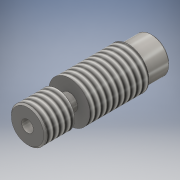
# Autodesk Inventor part: Heatbreak
Saved by Autodesk Inventor 2016 (Build 200138000, 138)
## iProperties
Created: 2016-03-26
Part Number: Heatbreak
Material: Stainless Steel
Document SubType Name: Modeling
Designer: Scott
Density: 8 g/cm^3
Appearance: Semi-Polished
Mass: 5.24058 g
Surface Area: 5.31118 cm^2
Volume: 0.655072 cm^3
Author: Scott
Autodesk Inventor part; units mm, degrees
ref_plane "YZ Plane" through (0, 0, 0) normal (1, 0, 0) x (0, 1, 0)
ref_plane "XZ Plane" through (0, 0, 0) normal (0, 1, 0) x (-1, 0, 0)
ref_plane "XY Plane" through (0, 0, 0) normal (0, 0, 1) x (1, 0, 0)
sketch "Sketch1" plane through (0, 0, 0) normal (0, 0, 1) x (1, 0, 0)
  line L0 (0, 0) -> (3, 0)
  line L1 (3, 0) -> (3, 5)
  line L2 (3, 5) -> (1.4, 5)
  line L3 (1.4, 5) -> (1.4, 7.1)
  line L4 (1.4, 7.1) -> (3.5, 7.1)
  line L5 (3.5, 7.1) -> (3.5, 17.1)
  line L6 (3.5, 17.1) -> (3, 17.1)
  line L7 (3, 17.1) -> (3, 21.2)
  line L8 (3, 21.2) -> (0, 21.2)
  line L9 (0, 21.2) -> (0, 0)
  dimension "d0" = 2.1
  dimension "d1" = 7.1
  dimension "d3" = 10
  dimension "d4" = 14.1
  dimension "d5" = 3
  dimension "d6" = 1.4
  dimension "d7" = 3.5
  dimension "d8" = 3
  constraints: 20 end point, 9 perpendicular, 1 horizontal
  measures "d0" distance between parallel lines of L4 L2
  measures "d1" distance between parallel lines of L0 L4
  measures "d3" distance of L4.end L5.end
  measures "d4" distance between parallel lines of L8 L4
  measures "d5" distance between parallel lines of L9 L1
  measures "d6" distance between parallel lines of L9 L3
  measures "d7" distance between parallel lines of L9 L5
  measures "d8" distance of L7.end L8.end
revolve "Revolution1" add sketch "Sketch1" angle 360 about axis through (0, 21.2, 0) along (0, -1, 0)
thread "Thread1" size "M7x1" class "6g" standard "ANSI Metric M Profile" full length
thread "Thread2" size "M6x1" class "6g" standard "ANSI Metric M Profile" full length
sketch "Sketch2" plane through (0, 21.2, 0) normal (0, 1, 0) x (1, 0, 0)
  circle A0 centre (0, 0) radius 3 projected
  point P0 (0, 0)
hole "Hole1" at (0, 21.2, 0) direction (0, -1, 0) diameter 2 end through all
hole "Hole2" at (0, 21.2, 0) direction (0, -1, 0) diameter 4.2 depth 5 tip angle 118
chamfer "Chamfer1" distance 0.25 angle 45 1 edges at (-3, 21.2, 0)
chamfer "Chamfer2" distance 0.25 angle 45 1 edges at (-3, 0, 0)
body "Solid1"
